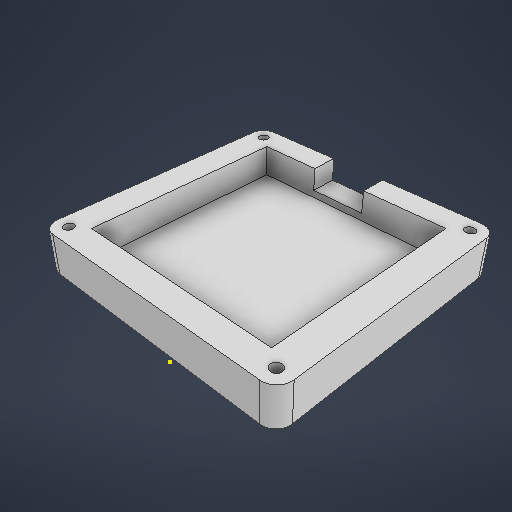
# Autodesk Inventor part: Case_Bottom
Saved by Autodesk Inventor 2026.1 (Build 301233000, 233)
## iProperties
Created: 2025-12-06
Part Number: Case_Bottom
Material: Generic
Document SubType Name: Modeling
Designer: chest
Density: 1 g/cm^3
Appearance: Default
Author: chest
Autodesk Inventor part; units mm, degrees
ref_plane "YZ Plane" through (0, 0, 0) normal (1, 0, 0) x (0, 1, 0)
ref_plane "XZ Plane" through (0, 0, 0) normal (0, 1, 0) x (-1, 0, 0)
ref_plane "XY Plane" through (0, 0, 0) normal (0, 0, 1) x (1, 0, 0)
sketch "Sketch1" plane through (0, 0, 0) normal (0, 1, 0) x (-1, 0, 0)
  line L0 (54.6183, -19.0153) -> (-12.4217, -19.0153)
  line L1 (-12.4217, -19.0153) -> (-12.4217, -83.5153)
  line L2 (-12.4217, -83.5153) -> (54.6183, -83.5153)
  line L3 (54.6183, -83.5153) -> (54.6183, -19.0153)
  line L4 (-21.9217, -9.5153) -> (64.1183, -9.5153)
  line L5 (64.1183, -9.5153) -> (64.1183, -93.0153)
  line L6 (64.1183, -93.0153) -> (-21.9217, -93.0153)
  line L7 (-21.9217, -93.0153) -> (-21.9217, -9.5153)
  circle A0 centre (-16.9217, -14.5153) radius 1.7
  circle A1 centre (-16.9217, -88.0153) radius 1.7
  circle A2 centre (59.1183, -88.0153) radius 1.7
  circle A3 centre (59.1183, -14.5153) radius 1.7
  circle A4 centre (59.1183, -14.5153) radius 3
  circle A5 centre (-16.9217, -14.5153) radius 3
  circle A6 centre (-16.9217, -88.0153) radius 3
  circle A7 centre (59.1183, -88.0153) radius 3
  point P0 (0, 0)
  point P1 (64.1183, -51.2653)
  dimension "d0" = 67.04
  dimension "d1" = 64.5
  dimension "d2" = 86.04
  dimension "d3" = 83.5
  dimension "d4" = 9.5
  dimension "d5" = 9.5
  dimension "d6" = 3.4
  dimension "d7" = 5
  dimension "d8" = 5
  dimension "d9" = 3.4
  dimension "d10" = 5
  dimension "d11" = 5
  dimension "d12" = 3.4
  dimension "d13" = 5
  dimension "d14" = 5
  dimension "d15" = 3.4
  dimension "d16" = 5
  dimension "d17" = 5
  dimension "d18" = 6
  dimension "d19" = 6
  dimension "d20" = 6
  dimension "d21" = 6
  constraints: 16 end point, 8 centre point, 4 coincident, 4 parallel, 2 horizontal, 2 perpendicular, 1 midpoint
  measures "d0" distance of L2.end L1.end
  measures "d1" distance of L1.end L0.end
  measures "d2" distance of L5.end L6.end
  measures "d3" distance of L4.end L5.end
  measures "d4" distance between parallel lines of L6 L2
  measures "d5" distance from line of point (64.118, -51.265) L3
  measures "d6" diameter of A0
  measures "d7" distance from line of L4 A0.centre
  measures "d8" distance from line of L7 A0.centre
  measures "d9" diameter of A1
  measures "d10" distance from line of L7 A1.centre
  measures "d11" distance from line of L6 A1.centre
  measures "d12" diameter of A2
  measures "d13" distance from line of L6 A2.centre
  measures "d14" distance from line of L5 A2.centre
  measures "d15" diameter of A3
  measures "d16" distance from line of L5 A3.centre
  measures "d17" distance from line of L4 A3.centre
  measures "d18" diameter of A4
  measures "d19" diameter of A5
  measures "d20" diameter of A6
  measures "d21" diameter of A7
extrude "Extrusion1" add sketch "Sketch1" along normal blind 13 contours L3 L2 L1 L0 | L4 L5 L6 L7 | A0 | A1 | A2 | A3 | A4 | A5 | A6 | A7
sketch "Sketch3" plane through (0, 13, 0) normal (0, 1, 0) x (1, 0, 0)
  circle A0 centre (-59.1183, 14.5153) radius 1.7
  line L0 (-64.1183, 9.5153) -> (21.9217, 9.5153) projected
  line L1 (-64.1183, 93.0153) -> (-64.1183, 9.5153) projected
  circle A1 centre (16.9217, 14.5153) radius 1.7
  line L2 (21.9217, 9.5153) -> (21.9217, 93.0153) projected
  circle A2 centre (16.9217, 88.0153) radius 1.7
  line L3 (21.9217, 93.0153) -> (-64.1183, 93.0153) projected
  circle A3 centre (-59.1183, 88.0153) radius 1.7
  point P0 (0, 0)
  dimension "d24" = 3.4
  dimension "d25" = 5
  dimension "d26" = 5
  dimension "d27" = 3.4
  dimension "d28" = 5
  dimension "d29" = 5
  dimension "d30" = 3.4
  dimension "d31" = 5
  dimension "d32" = 5
  dimension "d33" = 3.4
  dimension "d34" = 5
  dimension "d35" = 5
  constraints: 4 centre point
  measures "d24" diameter of A0
  measures "d25" distance from line of L0 A0.centre
  measures "d26" distance from line of A0.centre L1
  measures "d27" diameter of A1
  measures "d28" distance from line of L0 A1.centre
  measures "d29" distance from line of L2 A1.centre
  measures "d30" diameter of A2
  measures "d31" distance from line of L3 A2.centre
  measures "d32" distance from line of L2 A2.centre
  measures "d33" diameter of A3
  measures "d34" distance from line of L3 A3.centre
  measures "d35" distance from line of L1 A3.centre
extrude "Extrusion2" cut sketch "Sketch3" against normal blind 13 contours A0 | A1 | A2 | A3
sketch "Sketch6" plane through (0, 13, 0) normal (0, 1, 0) x (1, 0, 0)
  point P0 (0, 0)
sketch "Sketch7" plane through (0, 13, 0) normal (0, 1, 0) x (1, 0, 0)
  line L0 (21.9217, 93.0153) -> (-64.1183, 93.0153) projected
  line L1 (-54.1183, 84.2853) -> (11.9217, 84.2853)
  line L2 (21.9217, 9.5153) -> (21.9217, 93.0153) projected
  line L3 (-64.1183, 9.5153) -> (21.9217, 9.5153) projected
  line L4 (-21.0983, 18.2453) -> (-54.1183, 18.2453)
  line L5 (-21.0983, 18.2453) -> (11.9217, 18.2453)
  line L6 (-54.1183, 84.2853) -> (-54.1183, 18.2453)
  line L7 (11.9217, 18.2453) -> (11.9217, 84.2853)
  point P0 (0, 0)
  constraints: 10 end point, 1 parallel, 1 vertical
extrude "Extrusion3" cut sketch "Sketch7" against normal blind 10
fillet "Fillet1" radius 5 4 edges at (-64.1183, 6.5, -9.5153) (21.9217, 6.5, -9.5153) (21.9217, 6.5, -93.0153) (-64.1183, 6.5, -93.0153)
sketch "Sketch8" plane through (0, 13, 0) normal (0, 1, 0) x (1, 0, 0)
  line L0 (-54.1183, 84.2853) -> (11.9217, 84.2853) projected
  line L1 (16.9217, 93.0153) -> (-59.1183, 93.0153) projected
  line L2 (-34.1183, 84.2853) -> (-15.6183, 84.2853)
  line L3 (-15.6183, 84.2853) -> (-15.6183, 93.0153)
  line L4 (-15.6183, 93.0153) -> (-34.1183, 93.0153)
  line L5 (-34.1183, 93.0153) -> (-34.1183, 84.2853)
  line L6 (-64.1183, 88.0153) -> (-64.1183, 14.5153) projected
  point P0 (0, 0)
  dimension "d48" = 18.5
  dimension "d49" = 30
  constraints: 8 end point, 2 parallel, 2 point on line, 1 horizontal, 1 perpendicular
  measures "d48" distance of L4.end L3.end
  measures "d49" distance between parallel lines of L6 L5
extrude "Extrusion4" cut sketch "Sketch8" against normal blind 7.5
body "Solid1"
